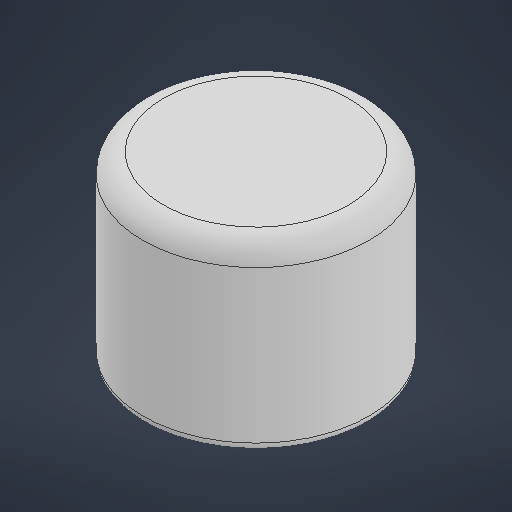
# Autodesk Inventor part: tapap
Saved by Autodesk Inventor 2026.1 (Build 301233020, 233B)
## iProperties
Created: 2025-12-13
Part Number: tapap
Material: Genérico
Document SubType Name: Modeling
Designer: anama
Density: 1 g/cm^3
Appearance: Valor por defecto
Author: anama
Autodesk Inventor part; units mm, degrees
ref_plane "YZ Plane" through (0, 0, 0) normal (1, 0, 0) x (0, 1, 0)
ref_plane "XZ Plane" through (0, 0, 0) normal (0, 1, 0) x (-1, 0, 0)
ref_plane "XY Plane" through (0, 0, 0) normal (0, 0, 1) x (1, 0, 0)
sketch "Boceto1" plane through (0, 0, 0) normal (0, 0, 1) x (1, 0, 0)
  circle A0 centre (0, 0) radius 13.5
  circle A1 centre (0, 0) radius 17.5
  line L0 (17.5, 1.27) -> (17.5, 24.003)
  line L1 (13.5, 1.27) -> (13.5, 20.828)
  line L2 (10.325, 24.003) -> (0, 24.003)
  line L3 (17.5, 24.003) -> (17.5, 24.828)
  line L4 (14.325, 28.003) -> (0, 28.003)
  line L5 (0, 28.003) -> (0, 0)
  arc A2 (17.5, 24.828) -> (14.325, 28.003) centre (14.325, 24.828) ccw
  arc A3 (13.5, 20.828) -> (10.325, 24.003) centre (10.325, 20.828) ccw
  line L6 (16.23, 0) -> (14.77, 0)
  arc A4 (16.23, 0) -> (17.5, 1.27) centre (16.23, 1.27) ccw
  arc A5 (13.5, 1.27) -> (14.77, 0) centre (14.77, 1.27) ccw
  point P0 (17.5, 0)
  point P1 (13.5, 0)
  point P2 (17.5, 28.003)
  dimension "d0" = 27
  dimension "d1" = 35
  dimension "d2" = 24.003
  dimension "d3" = 4
  dimension "d4" = 3.175
  dimension "d5" = 1.27
  constraints: 14 end point, 8 point on circle, 8 tangent, 6 point on line, 5 vertical, 4 centre point, 2 coincident, 2 equal radius, 2 horizontal alignment, 1 horizontal, 1 perpendicular, 4 other
  measures "d2" distance of point (17.5, 0) L0.end
  measures "d3" distance of L0.end point (17.5, 28.003)
  measures "d4" radius of A2
  measures "d5" radius of A4
revolve "Revolución1" add sketch "Boceto1" angle 360 about axis through (0, 28.003, 0) along (0, -1, 0) picked at (14.1771, 6.8232) contours L1 A3 L2 L5 L4 A2 L3 L0 A4 A1 | A1 A4 L6 A5 L1
